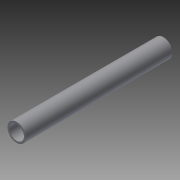
# Autodesk Inventor part: toptube
Saved by Autodesk Inventor 2015 (Build 190159000, 159)
## iProperties
Created: 2014-12-01
Part Number: toptube
Material: 常规
Document SubType Name: Modeling
Designer: zenkr
Density: 1 g/cm^3
Appearance: 默认
Author: zenkr
Autodesk Inventor part; units mm, degrees
ref_plane "YZ Plane" through (0, 0, 0) normal (1, 0, 0) x (0, 1, 0)
ref_plane "XZ Plane" through (0, 0, 0) normal (0, 1, 0) x (-1, 0, 0)
ref_plane "XY Plane" through (0, 0, 0) normal (0, 0, 1) x (1, 0, 0)
sketch "草图1" plane through (0, 0, 0) normal (0, 1, 0) x (-1, 0, 0)
  circle A0 centre (0, 0) radius 0.5
  dimension "d0" = 1
  constraints: 1 centre point, 1 coincident
  measures "d0" diameter of A0
extrude "拉伸1" add sketch "草图1" along normal blind 8
shell "抽壳1" thickness 0.1 removed faces 2 at (-0.3086, 0, -0.1558) at (-0.3086, 8, -0.1558)
